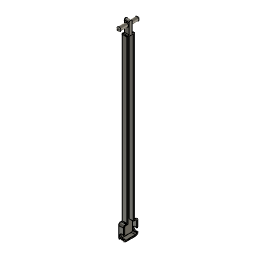
Connecting Rod (Autodesk Fusion 360 design; units mm, degrees)
Autodesk Fusion 360 part; units mm, degrees
sketch "Sketch1" plane through (0, 0, 0) normal (0, 1, 0) x (1, 0, 0)
  line L0 (-96.8714, -11.2087) -> (-103.8714, -11.2087)
  line L1 (-103.8714, -11.2087) -> (-103.8714, -246.2087)
  line L2 (-103.8714, -246.2087) -> (-96.8714, -246.2087)
  line L3 (-96.8714, -246.2087) -> (-96.8714, -11.2087)
  dimension "d145" = 7
  dimension "d146" = 235
  constraint horizontal L0
  constraint vertical L1
  constraint horizontal L2
  constraint vertical L3
  measures "d145" distance of L1 L3
  measures "d146" distance of L0 L2
extrude "Extrude1" add sketch "Sketch1" along normal mid plane 10
sketch "Sketch2" plane through (-103.8714, 0, 0) normal (-1, 0, 0) x (0, -1, 0)
  line L0 (-9.5, 31.2087) -> (9.5, 31.2087)
  line L1 (9.5, 31.2087) -> (9.5, 11.2087)
  line L2 (9.5, 11.2087) -> (-9.5, 11.2087)
  line L3 (-9.5, 11.2087) -> (-9.5, 31.2087)
  line L4 (-7.5, 20.7119) -> (-7.5, 27.7217)
  line L5 (7.5, 27.7217) -> (7.5, 20.7119)
  line L6 (5, 11.2087) -> (-5, 11.2087)
  dimension "d149" = 2
  dimension "d150" = 2
  dimension "d151" = 20
  constraint horizontal L0
  constraint vertical L1
  constraint horizontal L2
  constraint vertical L3
  constraint collinear L2 L6
  measures "d149" distance of L3 L4
  measures "d150" distance of L1 L5
  measures "d151" distance of L0 L2
extrude "Extrude2" add sketch "Sketch2" against normal up to surface (7 mm away)
fillet "Fillet1" radius 3 4 edges at (-100.3714, 9.5, 11.2087) (-100.3714, 9.5, 31.2087) (-100.3714, -9.5, 11.2087) (-100.3714, -9.5, 31.2087)
shell "Shell1" thickness 1.5 removed faces 1 at (-96.8714, -1.6667, 19.8753)
sketch "Sketch3" plane through (0, 0, 0) normal (0, 1, 0) x (1, 0, 0)
  circle A0 centre (-98.8714, -17.4087) radius 3
  line L0 (-96.8714, -11.2087) -> (-96.8714, -14.2087)
  line L1 (-96.8714, -11.2087) -> (-103.8714, -11.2087)
  point P0 (-96.8714, -11.2087)
  dimension "d159" = 6
  dimension "d160" = 2
  dimension "d161" = 6.2
  measures "d159" diameter of A0
  measures "d160" distance of A0.centre L0
  measures "d161" vertical distance of A0.centre P0
extrude "Extrude3" cut sketch "Sketch3" along normal through all and the other way through all
sketch "Sketch4" plane through (0, 0, 246.2087) normal (0, 0, 1) x (-1, 0, 0)
  line L0 (103.8714, -2) -> (96.8714, -2)
  line L1 (96.8714, -2) -> (96.8714, 2)
  line L2 (96.8714, 2) -> (103.8714, 2)
  line L3 (103.8714, 2) -> (103.8714, -2)
  line L4 (103.8714, 5) -> (103.8714, -5)
  line L5 (96.8714, -5) -> (96.8714, 5)
  line L6 (103.8714, -5) -> (96.8714, -5)
  line L7 (96.8714, 5) -> (103.8714, 5)
  dimension "d163" = 3
  dimension "d164" = 3
  constraint horizontal L0
  constraint vertical L1
  constraint horizontal L2
  constraint vertical L3
  constraint coincident L1.end L5
  constraint coincident L0.start L4
  measures "d163" distance of L0 L6
  measures "d164" distance of L2 L7
extrude "Extrude4" add sketch "Sketch4" along normal blind 16 contours L0 L1 L2 L3 L4 L5
fillet "Fillet4" radius 2 2 edges at (-100.3714, 2, 262.2087) (-100.3714, -2, 262.2087)
sketch "Sketch5" plane through (0, 0, 0) normal (0, 1, 0) x (1, 0, 0)
  circle A0 centre (-100.3714, -256.2087) radius 2.5
  line L0 (-103.8714, -246.2087) -> (-96.8714, -246.2087)
  line L1 (-103.8714, -246.2087) -> (-103.8714, -260.2087)
  dimension "d168" = 5
  dimension "d169" = 10
  dimension "d170" = 3.5
  measures "d168" diameter of A0
  measures "d169" distance of A0.centre L0
  measures "d170" distance of A0.centre L1
extrude "Extrude5" add sketch "Sketch5" along normal mid plane 28
fillet "Fillet5" radius 2 2 edges at (-102.7022, 14, 257.1127) (-102.7022, -14, 255.3046)
fillet "Fillet6" radius 0.8 18 edges at (-103.8714, 5, 138.7087) (-103.8714, -5, 138.7087) (-103.8714, -5.75, 31.2087) (-103.8714, -8.6213, 30.33) (-103.8714, -9.5, 21.2087) (-103.8714, -8.6213, 12.0873) (-103.8714, 0, 11.2087) (-103.8714, 8.6213, 12.0873) (-103.8714, 9.5, 21.2087) (-103.8714, 8.6213, 30.33) (-103.8714, 5.75, 31.2087) (-103.8714, 3.5, 246.2087) (-103.8714, 2, 253.2087) (-103.8714, 0, 262.2087) (-103.8714, -2, 253.2087) (-103.8714, -3.5, 246.2087) (-100.3714, 5, 246.2087) (-100.3714, -5, 246.2087)
